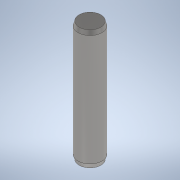
# Autodesk Inventor part: f2w10
Saved by Autodesk Inventor 2020 (Build 240168000, 168)
## iProperties
Created: 2020-03-24
Part Number: f2w10
Material: ステンレス鋼
Document SubType Name: Modeling
Designer: happy
Density: 8 g/cm^3
Appearance: 半つや出し
Mass: 0.249729 g
Surface Area: 0.679334 cm^2
Volume: 0.0312161 cm^3
Author: happy
## iProperties of the stored document _3D プリント.ipt
Created: 2020-06-15
Part Number: _3D プリント
Material: 一般
Document SubType Name: Modeling
Designer: happy
Density: 1 g/cm^3
Appearance: 既定
Author: happy
Autodesk Inventor part; units mm, degrees
ref_plane "YZ Plane" through (0, 0, 0) normal (1, 0, 0) x (0, 1, 0)
ref_plane "XZ Plane" through (0, 0, 0) normal (0, 1, 0) x (-1, 0, 0)
ref_plane "XY Plane" through (0, 0, 0) normal (0, 0, 1) x (1, 0, 0)
sketch "スケッチ2" plane through (0, 0, 0) normal (1, 0, 0) x (0, 1, 0)
  line L0 (5, 1) -> (-5, 1)
  line L1 (-5, 1) -> (-5, -1)
  line L2 (-5, -1) -> (5, -1)
  line L3 (5, -1) -> (5, 1)
  line L4 (5, 1) -> (-5, -1) construction
  line L5 (-5, 1) -> (5, -1) construction
  line L6 (5, -0.9062) -> (4.65, -1)
  line L7 (5, 0) -> (-5, 0)
  line L8 (-4.65, -1) -> (-5, -0.9062)
  point P0 (0, 0)
  dimension "d9" = 10
  dimension "d10" = 2
  dimension "d11" = 0.35
  dimension "d12" = 15
  dimension "d14" = 0.35
  dimension "d15" = 15
  constraints: 18 end point, 4 midpoint, 4 point on line, 2 parallel, 1 horizontal, 1 perpendicular
  measures "d9" distance of L2.end L1.end
  measures "d10" distance of L1.end L0.end
  measures "d11" distance of L6.end L2.end
  measures "d12" angle of L6 L2
  measures "d14" distance of L1.end L8.start
  measures "d15" angle of L2 L8
revolve "回転1" add sketch "スケッチ2" angle 360 about axis through (0, 5, 0) along (0, -1, 0) contours L3 L6 L2 L8 L1 L7
